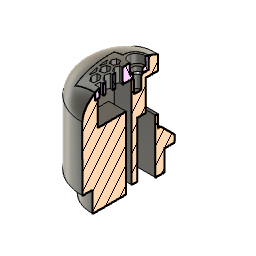
sensorhead_v2_filterBolt v4 (Autodesk Fusion 360 design; units mm, degrees)
Autodesk Fusion 360 part; units mm, degrees
sketch "Sketch1" plane through (0, 0, 0) normal (0, 0, 1) x (1, 0, 0)
  circle A0 centre (0, 0) radius 13
  dimension "d1" = 26
  constraint coincident A0.centre origin
  measures "d1" diameter of A0
extrude "Extrude1" add sketch "Sketch1" along normal blind 7.5 makes body 1
sketch "Sketch2" plane through (0, 0, 7.5) normal (0, 0, 1) x (-1, 0, 0)
  circle A0 centre (0, 0) radius 13
  circle A1 centre (0, 0) radius 16.7
  dimension "d4" = 33.4
  constraint coincident A0.centre A1.centre
  measures "d4" diameter of A1
extrude "Extrude2" add sketch "Sketch2" along normal blind 30 contours A0 | A1 bodies 1
sketch "Sketch8" plane through (0, 0, 0) normal (0, 1, 0) x (1, 0, 0)
  line L0 (0, -37.5) -> (0, -27.5)
  line L1 (16.7, -27.5) -> (0, -27.5)
  line L2 (0, -27.5) -> (0, -37.5)
  ellipse E0 centre (0, -27.5) end of major axis (-16.7, -27.5) minor radius 10 (0, -37.5) -> (16.7, -27.5) ccw
  line L3 (16.7, -27.5) -> (16.7, -37.5)
  line L4 (16.7, -37.5) -> (0, -37.5)
  dimension "d66" = 10
  dimension "d67" = 33.4
  constraint vertical L0
  constraint coincident L0.end L1.end
  constraint perpendicular L1 L3
  constraint perpendicular L3 L4
  measures "d66" distance of L0.start L0.end
  measures "d67" distance of E0
revolve "Revolve1" cut sketch "Sketch8" angle 360 about axis through (0, 0, 27.5) along (0, 0, 1) contours E0 L3 L4 bodies 1
sketch "Sketch3" plane through (0, 0, 0) normal (0, 0, -1) x (1, 0, 0)
  circle A0 centre (0, 0) radius 13
  line L0 (-7.875, -6.2) -> (7.875, -6.2)
  line L1 (7.875, -6.2) -> (7.875, -8.2)
  line L2 (-7.875, -8.2) -> (-7.875, -6.2)
  line L3 (-7.875, -6.2) -> (7.875, -8.2) construction
  line L4 (7.875, -6.2) -> (-7.875, -8.2) construction
  line L5 (6.5, -8.2) -> (6.5, -9.7)
  line L6 (-6.5, -9.7) -> (-6.5, -8.2)
  line L7 (-6.5, -8.2) -> (6.5, -10.2) construction
  line L8 (6.5, -8.2) -> (-6.5, -10.2) construction
  line L9 (-6.5, -6.2) -> (6.5, -6.2)
  line L10 (6.5, -6.2) -> (6.5, -1.2)
  line L11 (6.5, -1.2) -> (-6.5, -1.2)
  line L12 (-6.5, -1.2) -> (-6.5, -6.2)
  line L13 (-6.5, -6.2) -> (6.5, -1.2) construction
  line L14 (6.5, -6.2) -> (-6.5, -1.2) construction
  line L15 (7.875, -8.2) -> (6.5, -8.2)
  line L16 (-6.5, -8.2) -> (-7.875, -8.2)
  line L17 (6.5, -9.7) -> (-6.5, -9.7)
  point P0 (0, -7.2)
  point P1 (0, -9.2)
  point P2 (0, -3.7)
  dimension "d9" = 15.75
  dimension "d10" = 2
  dimension "d13" = 13
  dimension "d15" = 13
  dimension "d132" = 0.5
  constraint horizontal L0
  constraint perpendicular L0 L1
  constraint parallel L0 L15
  constraint parallel L1 L2
  constraint coincident L3 P0
  constraint coincident L4 P0
  constraint parallel L5 L6
  constraint coincident L7 P1
  constraint coincident L8 P1
  constraint horizontal L9
  constraint perpendicular L9 L10
  constraint parallel L9 L11
  constraint parallel L10 L12
  constraint coincident L13 P2
  constraint coincident L14 P2
  constraint collinear L15 L16
  constraint perpendicular L6 L17
  measures "d9" distance of L1.end L2.start
  measures "d10" distance of L0.end L1.end
  measures "d13" distance of L7.end L8.end
  measures "d15" distance of L10.end L11.end
  measures "d132" distance of L7.end L5.end
sketch "Sketch4" plane through (0, 0, 0) normal (1, 0, 0) x (0, 1, 0)
  line L0 (0, 12) -> (10.7, 12)
  line L1 (10.7, 12) -> (21.5887, 12)
  line L2 (21.5887, 12) -> (21.5887, 38.7585)
  line L3 (21.5887, 38.7585) -> (10.7, 38.7585)
  line L4 (10.7, 38.7585) -> (10.7, 12)
  dimension "d17" = 10.7
  constraint horizontal L1
  constraint vertical L2
  constraint horizontal L3
  constraint vertical L4
  measures "d17" distance of L0.start L0.end
sketch "Sketch5" plane through (0, 0, 0) normal (1, 0, 0) x (0, 1, 0)
extrude "Extrude3" cut sketch "Sketch4" along normal blind 26 bodies 1
extrude "Extrude4" cut 1 faces at (0, 12.7, 24.8926) along direction (-1, 0, 0) blind 20 on bodies 1 bodies 1
extrude "Extrude5" cut sketch "Sketch3" against normal blind 30 contours L0 L1 L2 L5 L6 L9 L15 L16 L17 bodies 1
extrude "Extrude6" cut sketch "Sketch3" against normal blind 19 contours L0 L9 L10 L11 L12 bodies 1
sketch "Sketch6" plane through (0, 10.7, 0) normal (0, 1, 0) x (-1, 0, 0)
  line L0 (-12.8219, 27.5) -> (-12.8219, 12)
  line L1 (-12.8219, 12) -> (12.8219, 12)
  line L2 (6.5, 16.5) -> (-6.5, 16.5)
  line L3 (-6.5, 16.5) -> (-6.5, 29.5)
  line L4 (-6.5, 29.5) -> (6.5, 29.5)
  line L5 (6.5, 29.5) -> (6.5, 16.5)
  line L6 (6.5, 16.5) -> (-6.5, 29.5) construction
  line L7 (-6.5, 16.5) -> (6.5, 29.5) construction
  line L8 (12.8219, 12) -> (12.8219, 27.5)
  spline S0 degree 3 poles (0, 35.1778) (0.2245, 35.1778) (0.4491, 35.1742) (1.1338, 35.1527) (1.5943, 35.1233) (2.7541, 35.0106) (3.4543, 34.9068) (5.6711, 34.4534) (7.1958, 33.9489) (9.6653, 32.6226) (10.586, 31.9216) (11.7837, 30.5905) (12.1987, 29.9679) (12.6993, 28.7104) (12.8219, 28.1132) (12.8219, 27.5) knots -1.453792 -1.453792 -1.453792 -1.453792 -1.397904 -1.397904 -1.283214 -1.283214 -1.107738 -1.107738 -0.719665 -0.719665 -0.405775 -0.405775 -0.183953 -0.183953 0 0 0 0
  spline S1 degree 3 poles (-12.8219, 27.5) (-12.8219, 27.8392) (-12.7843, 28.1754) (-12.6354, 28.8496) (-12.5226, 29.1821) (-12.055, 30.2186) (-11.5805, 30.8593) (-10.1007, 32.3522) (-8.8544, 33.1585) (-6.5098, 34.1443) (-5.6112, 34.4282) (-3.9195, 34.8277) (-3.1196, 34.963) (-1.813, 35.1068) (-1.3053, 35.1439) (-0.532, 35.1728) (-0.266, 35.1778) (0, 35.1778) knots -1.833651 -1.833651 -1.833651 -1.833651 -1.708322 -1.708322 -1.578523 -1.578523 -1.288251 -1.288251 -0.803835 -0.803835 -0.524093 -0.524093 -0.282154 -0.282154 -0.129741 -0.129741 -0.04999 -0.04999 -0.04999 -0.04999
  point P0 (0, 23)
  dimension "d26" = 13
  dimension "d27" = 13
  constraint horizontal L2
  constraint perpendicular L2 L3
  constraint parallel L2 L4
  constraint parallel L3 L5
  constraint coincident L6 P0
  constraint coincident L7 P0
  measures "d26" distance of L3.end L4.end
  measures "d27" distance of L2.end L3.end
extrude "Extrude7" cut sketch "Sketch6" against normal blind 1 contours L2 L3 L4 L5 bodies 1
extrude "Extrude8" cut 1 faces at (2.1667, 10.3667, 29.5) along direction (0, 0, 1) blind 0.5 on bodies 1 bodies 1
ref_plane "WorkPlane1" through (0, 0, 40) normal (0, 0, 1) x (1, 0, 0)
sketch "Sketch7" plane through (0, 0, 40) normal (0, 0, 1) x (1, 0, 0)
  line L0 (7, 2) -> (7, -12)
  line L1 (7, -12) -> (-7, -12)
  line L2 (-7, -12) -> (-7, 2)
  line L3 (-7, 2) -> (7, -12) construction
  line L4 (7, 2) -> (-7, -12) construction
  line L5 (7.125, 2.125) -> (7.125, -12.125)
  line L6 (7.125, -12.125) -> (-7.125, -12.125)
  line L7 (-7.125, -12.125) -> (-7.125, 2.125)
  line L8 (-7.125, 2.125) -> (7.125, -12.125) construction
  line L9 (7.125, 2.125) -> (-7.125, -12.125) construction
  line L10 (-4, 2.125) -> (-4, 3.325)
  line L11 (4, 2.125) -> (4, 3.325)
  line L12 (-7.125, 2.125) -> (-4, 2.125)
  line L13 (4, 2.125) -> (7.125, 2.125)
  arc A0 (4, 3.325) -> (-4, 3.325) centre (0, 3.325) ccw
  line L14 (-4, 2) -> (-3.9, 2)
  line L15 (-3.9, 2) -> (-3.9, 3.325)
  line L16 (4, 2) -> (3.9, 2)
  line L17 (3.9, 2) -> (3.9, 3.325)
  arc A1 (3.9, 3.325) -> (-3.9, 3.325) centre (0, 3.325) ccw
  line L18 (-7, 2) -> (-3.9, 2)
  line L19 (3.9, 2) -> (7, 2)
  circle A2 centre (0, 3.325) radius 1.35
  circle A3 centre (0, 3.325) radius 2.1
  circle A4 centre (0, 3.325) radius 1.75
  circle A5 centre (0, 3.325) radius 2.875
  point P0 (0, -5)
  point P1 (0, -5)
  dimension "d35" = 14.25
  dimension "d36" = 14.25
  dimension "d135" = 7.8
  dimension "d136" = 0.1
  dimension "d137" = 0.1
  dimension "d138" = 2.7
  dimension "d139" = 4.2
  dimension "d140" = 3.5
  dimension "d141" = 5.75
  constraint horizontal L18
  constraint perpendicular L0 L18
  constraint parallel L1 L18
  constraint parallel L0 L2
  constraint coincident L3 P1
  constraint coincident L4 P1
  constraint horizontal L12
  constraint perpendicular L5 L12
  constraint parallel L6 L12
  constraint parallel L5 L7
  constraint coincident L8 P1
  constraint coincident L9 P1
  constraint coincident P1 P0
  constraint vertical L10
  constraint collinear L12 L13
  constraint concentric A0 A1
  constraint coincident L14.start L18
  constraint parallel L14 L18
  constraint tangent L15 A1
  constraint perpendicular L15 L18
  constraint coincident L16.start L18
  constraint perpendicular L11 L16
  constraint vertical L17
  constraint tangent L17 A1
  constraint collinear L18 L19
  constraint concentric A0 A2
  constraint concentric A1 A3
  constraint concentric A2 A4
  constraint concentric A2 A5
  measures "d35" distance of L5.end L6.end
  measures "d36" distance of L5.start L5.end
  measures "d135" diameter of A1
  measures "d136" distance of L14.start L14.end
  measures "d137" distance of L16.start L16.end
  measures "d138" diameter of A2
  measures "d139" diameter of A3
  measures "d140" diameter of A4
  measures "d141" diameter of A5
copy_body "Body->Comp1" bodies 1 removing the originals makes body 2 in component "sensorHead"
extrude "Extrude11" add 1 faces at (15.4266, 0, 7.5) along direction (0, 0, -1) blind 3 on bodies 2 bodies 2 in component "sensorHead"
sketch "Sketch2 (2)" plane through (0, 0, 0) normal (1, 0, 0) x (0, 1, 0) in component "sensorHead"
  line L0 (10.7, 12) -> (16.7, 12)
  line L1 (-16.7, 4.5) -> (16.7, 4.5)
  line L2 (16.7, 12) -> (16.7, 4.5)
  line L3 (10.7, 12) -> (11.7, 12)
  line L4 (11.7, 12) -> (16.7, 7)
  line L5 (16.7, 12) -> (11.7, 12)
  point P0 (10.7, 12)
  dimension "d157" = 1
  dimension "d158" = 45
  constraint coincident L0.end L2.start
  constraint coincident L1.end L2.end
  constraint coincident P0 L0.start
  constraint coincident L0 L3.end
  constraint coincident L2 L4.end
  measures "d157" distance of P0 L3.end
  measures "d158" angle of L3 L4
extrude "Extrude5'" cut sketch "Sketch2 (2)" along normal mid plane 33 bodies 2 in component "sensorHead"
extrude "Extrude12" add 1 faces at (0.3238, -3.5212, 0) along direction (0, 0, -1) blind 3 on bodies 2 bodies 2 in component "sensorHead"
extrude "Extrude1'" cut sketch "Sketch7" against normal blind 8 contours L0 L1 L2 L14 L15 L16 L17 A1 L18 L19 | L5 L6 L7 L10 L11 L12 L13 A0 | A2 | A3 | A4 | A5 bodies 2 in component "sensorHead"
sketch "Sketch1 (2)" plane through (0, 0, 32) normal (0, 0, 1) x (-1, 0, 0) in component "sensorHead"
  line L0 (7.125, 12.125) -> (-7.125, 12.125)
  line L1 (-7.125, 12.125) -> (-7.125, -2.125)
  line L2 (4, -2.125) -> (7.125, -2.125)
  line L3 (7.125, -2.125) -> (7.125, 12.125)
  line L4 (6.125, -1.125) -> (-6.125, -1.125)
  line L5 (-6.125, -1.125) -> (-6.125, 11.125)
  line L6 (-6.125, 11.125) -> (6.125, 11.125)
  line L7 (6.125, 11.125) -> (6.125, -1.125)
  line L8 (6.125, -1.125) -> (-6.125, 11.125) construction
  line L9 (-6.125, -1.125) -> (6.125, 11.125) construction
  line L10 (-6.125, -1.125) -> (6.125, -1.125)
  line L11 (6.125, -1.125) -> (6.125, 0.875)
  line L12 (6.125, 0.875) -> (-6.125, 0.875)
  line L13 (-6.125, 0.875) -> (-6.125, -1.125)
  arc A0 (-4, -3.325) -> (4, -3.325) centre (0, -3.325) ccw
  line L14 (4, -3.325) -> (4, -2.125)
  line L15 (-7.125, -2.125) -> (-4, -2.125)
  line L16 (-4, -2.125) -> (-4, -3.325)
  point P0 (0, 5)
  dimension "d39" = 12.25
  dimension "d40" = 12.25
  dimension "d41" = 12.25
  dimension "d42" = 2
  constraint horizontal L4
  constraint perpendicular L4 L5
  constraint parallel L4 L6
  constraint parallel L5 L7
  constraint coincident L8 P0
  constraint coincident L9 P0
  constraint horizontal L10
  constraint vertical L11
  constraint horizontal L12
  constraint vertical L13
  measures "d39" distance of L5.end L6.end
  measures "d40" distance of L4.end L5.end
  measures "d41" distance of L4.end L4.start
  measures "d42" distance of L4.end L12.end
extrude "Extrude2'" cut sketch "Sketch1 (2)" against normal blind 47 contours L4 L5 L7 L10 L11 L12 L13 bodies 2 in component "sensorHead"
extrude "Extrude3'" add 2 faces at (2.1667, 1.2, -1) (2.1667, 1.2, 6.3333) along direction (0, 1, 0) blind 1.925 on bodies 2 bodies 2 in component "sensorHead"
extrude "Extrude4'" cut sketch "Sketch1 (2)" against normal blind 6 contours L5 L6 L7 L12 bodies 2 in component "sensorHead"
extrude "Extrude9" add sketch "Sketch7" against normal blind 7.9 separate body contours L0 L1 L2 L14 L15 L16 L17 A1 L18 L19 | A2 | A3 | A4 | A5 makes body 3
revolve "Revolve2" cut sketch "Sketch8" angle 360 about axis through (0, 0, 37.5) along (0, 0, -1) contours L0 L1 L2 E0 keep common part bodies 3
sketch "Sketch9" plane through (0, 0, 32.1) normal (0, 0, -1) x (1, 0, 0)
  line L0 (7, 12) -> (-7, 12)
  line L1 (-7, 12) -> (-7, -2)
  line L2 (3.9, -2) -> (7, -2)
  line L3 (7, -2) -> (7, 12)
  line L4 (7, -2) -> (-7, -2)
  line L5 (-7, -2) -> (-7, 12)
  line L6 (-7, 12) -> (7, 12)
  line L7 (7, 12) -> (7, -2)
  line L8 (-5.5, 10.5) -> (5.5, 10.5)
  line L9 (5.5, 10.5) -> (5.5, -0.5)
  line L10 (5.5, -0.5) -> (-5.5, -0.5)
  line L11 (-5.5, -0.5) -> (-5.5, 10.5)
  line L12 (1.5, -0.0043) -> (0.7537, 1.2969)
  line L13 (0.7537, 1.2969) -> (-0.7463, 1.3012)
  line L14 (-0.7463, 1.3012) -> (-1.5, 0.0043)
  line L15 (-1.5, 0.0043) -> (-0.7537, -1.2969)
  line L16 (-0.7537, -1.2969) -> (0.7463, -1.3012)
  line L17 (0.7463, -1.3012) -> (1.5, -0.0043)
  line L18 (-5.2537, -1.3012) -> (-4.5, -0.0043)
  line L19 (-6.7537, -1.2969) -> (-5.2537, -1.3012)
  line L20 (-7.5, 0.0043) -> (-6.7537, -1.2969)
  line L21 (-6.7463, 1.3012) -> (-7.5, 0.0043)
  line L22 (-5.2463, 1.2969) -> (-6.7463, 1.3012)
  line L23 (-4.5, -0.0043) -> (-5.2463, 1.2969)
  line L24 (6.7463, -1.3012) -> (7.5, -0.0043)
  line L25 (5.2463, -1.2969) -> (6.7463, -1.3012)
  line L26 (4.5, 0.0043) -> (5.2463, -1.2969)
  line L27 (5.2537, 1.3012) -> (4.5, 0.0043)
  line L28 (6.7537, 1.2969) -> (5.2537, 1.3012)
  line L29 (7.5, -0.0043) -> (6.7537, 1.2969)
  line L30 (-5.2537, 2.1988) -> (-4.5, 3.4957)
  line L31 (-6.7537, 2.2031) -> (-5.2537, 2.1988)
  line L32 (-7.5, 3.5043) -> (-6.7537, 2.2031)
  line L33 (-6.7463, 4.8012) -> (-7.5, 3.5043)
  line L34 (-5.2463, 4.7969) -> (-6.7463, 4.8012)
  line L35 (-4.5, 3.4957) -> (-5.2463, 4.7969)
  line L36 (0.7463, 2.1988) -> (1.5, 3.4957)
  line L37 (-0.7537, 2.2031) -> (0.7463, 2.1988)
  line L38 (-1.5, 3.5043) -> (-0.7537, 2.2031)
  line L39 (-0.7463, 4.8012) -> (-1.5, 3.5043)
  line L40 (0.7537, 4.7969) -> (-0.7463, 4.8012)
  line L41 (1.5, 3.4957) -> (0.7537, 4.7969)
  line L42 (6.7463, 2.1988) -> (7.5, 3.4957)
  line L43 (5.2463, 2.2031) -> (6.7463, 2.1988)
  line L44 (4.5, 3.5043) -> (5.2463, 2.2031)
  line L45 (5.2537, 4.8012) -> (4.5, 3.5043)
  line L46 (6.7537, 4.7969) -> (5.2537, 4.8012)
  line L47 (7.5, 3.4957) -> (6.7537, 4.7969)
  line L48 (-5.2537, 5.6988) -> (-4.5, 6.9957)
  line L49 (-6.7537, 5.7031) -> (-5.2537, 5.6988)
  line L50 (-7.5, 7.0043) -> (-6.7537, 5.7031)
  line L51 (-6.7463, 8.3012) -> (-7.5, 7.0043)
  line L52 (-5.2463, 8.2969) -> (-6.7463, 8.3012)
  line L53 (-4.5, 6.9957) -> (-5.2463, 8.2969)
  line L54 (0.7463, 5.6988) -> (1.5, 6.9957)
  line L55 (-0.7537, 5.7031) -> (0.7463, 5.6988)
  line L56 (-1.5, 7.0043) -> (-0.7537, 5.7031)
  line L57 (-0.7463, 8.3012) -> (-1.5, 7.0043)
  line L58 (0.7537, 8.2969) -> (-0.7463, 8.3012)
  line L59 (1.5, 6.9957) -> (0.7537, 8.2969)
  line L60 (6.7463, 5.6988) -> (7.5, 6.9957)
  line L61 (5.2463, 5.7031) -> (6.7463, 5.6988)
  line L62 (4.5, 7.0043) -> (5.2463, 5.7031)
  line L63 (5.2537, 8.3012) -> (4.5, 7.0043)
  line L64 (6.7537, 8.2969) -> (5.2537, 8.3012)
  line L65 (7.5, 6.9957) -> (6.7537, 8.2969)
  line L66 (-5.2537, 9.1988) -> (-4.5, 10.4957)
  line L67 (-6.7537, 9.2031) -> (-5.2537, 9.1988)
  line L68 (-7.5, 10.5043) -> (-6.7537, 9.2031)
  line L69 (-6.7463, 11.8012) -> (-7.5, 10.5043)
  line L70 (-5.2463, 11.7969) -> (-6.7463, 11.8012)
  line L71 (-4.5, 10.4957) -> (-5.2463, 11.7969)
  line L72 (0.7463, 9.1988) -> (1.5, 10.4957)
  line L73 (-0.7537, 9.2031) -> (0.7463, 9.1988)
  line L74 (-1.5, 10.5043) -> (-0.7537, 9.2031)
  line L75 (-0.7463, 11.8012) -> (-1.5, 10.5043)
  line L76 (0.7537, 11.7969) -> (-0.7463, 11.8012)
  line L77 (1.5, 10.4957) -> (0.7537, 11.7969)
  line L78 (6.7463, 9.1988) -> (7.5, 10.4957)
  line L79 (5.2463, 9.2031) -> (6.7463, 9.1988)
  line L80 (4.5, 10.5043) -> (5.2463, 9.2031)
  line L81 (5.2537, 11.8012) -> (4.5, 10.5043)
  line L82 (6.7537, 11.7969) -> (5.2537, 11.8012)
  line L83 (7.5, 10.4957) -> (6.7537, 11.7969)
  line L84 (3.7463, -3.2012) -> (4.5, -1.9043)
  line L85 (4.5, -1.9043) -> (3.7537, -0.6031)
  line L86 (3.7537, -0.6031) -> (2.2537, -0.5988)
  line L87 (2.2537, -0.5988) -> (1.5, -1.8957)
  line L88 (1.5, -1.8957) -> (2.2463, -3.1969)
  line L89 (2.2463, -3.1969) -> (3.7463, -3.2012)
  line L90 (-1.5, -1.9043) -> (-2.2463, -0.6031)
  line L91 (-2.2463, -0.6031) -> (-3.7463, -0.5988)
  line L92 (-3.7463, -0.5988) -> (-4.5, -1.8957)
  line L93 (-4.5, -1.8957) -> (-3.7537, -3.1969)
  line L94 (-3.7537, -3.1969) -> (-2.2537, -3.2012)
  line L95 (-2.2537, -3.2012) -> (-1.5, -1.9043)
  line L96 (-7.5, -1.9043) -> (-8.2463, -0.6031)
  line L97 (-8.2463, -0.6031) -> (-9.7463, -0.5988)
  line L98 (-9.7463, -0.5988) -> (-10.5, -1.8957)
  line L99 (-10.5, -1.8957) -> (-9.7537, -3.1969)
  line L100 (-9.7537, -3.1969) -> (-8.2537, -3.2012)
  line L101 (-8.2537, -3.2012) -> (-7.5, -1.9043)
  line L102 (4.5, 1.6582) -> (3.7537, 2.9594)
  line L103 (3.7537, 2.9594) -> (2.2537, 2.9637)
  line L104 (2.2537, 2.9637) -> (1.5, 1.6668)
  line L105 (1.5, 1.6668) -> (2.2463, 0.3656)
  line L106 (2.2463, 0.3656) -> (3.7463, 0.3613)
  line L107 (3.7463, 0.3613) -> (4.5, 1.6582)
  line L108 (-1.5, 1.6582) -> (-2.2463, 2.9594)
  line L109 (-2.2463, 2.9594) -> (-3.7463, 2.9637)
  line L110 (-3.7463, 2.9637) -> (-4.5, 1.6668)
  line L111 (-4.5, 1.6668) -> (-3.7537, 0.3656)
  line L112 (-3.7537, 0.3656) -> (-2.2537, 0.3613)
  line L113 (-2.2537, 0.3613) -> (-1.5, 1.6582)
  line L114 (-7.5, 1.6582) -> (-8.2463, 2.9594)
  line L115 (-8.2463, 2.9594) -> (-9.7463, 2.9637)
  line L116 (-9.7463, 2.9637) -> (-10.5, 1.6668)
  line L117 (-10.5, 1.6668) -> (-9.7537, 0.3656)
  line L118 (-9.7537, 0.3656) -> (-8.2537, 0.3613)
  line L119 (-8.2537, 0.3613) -> (-7.5, 1.6582)
  line L120 (4.5, 5.2207) -> (3.7537, 6.5219)
  line L121 (3.7537, 6.5219) -> (2.2537, 6.5262)
  line L122 (2.2537, 6.5262) -> (1.5, 5.2293)
  line L123 (1.5, 5.2293) -> (2.2463, 3.9281)
  line L124 (2.2463, 3.9281) -> (3.7463, 3.9238)
  line L125 (3.7463, 3.9238) -> (4.5, 5.2207)
  line L126 (-1.5, 5.2207) -> (-2.2463, 6.5219)
  line L127 (-2.2463, 6.5219) -> (-3.7463, 6.5262)
  line L128 (-3.7463, 6.5262) -> (-4.5, 5.2293)
  line L129 (-4.5, 5.2293) -> (-3.7537, 3.9281)
  line L130 (-3.7537, 3.9281) -> (-2.2537, 3.9238)
  line L131 (-2.2537, 3.9238) -> (-1.5, 5.2207)
  line L132 (-7.5, 5.2207) -> (-8.2463, 6.5219)
  line L133 (-8.2463, 6.5219) -> (-9.7463, 6.5262)
  line L134 (-9.7463, 6.5262) -> (-10.5, 5.2293)
  line L135 (-10.5, 5.2293) -> (-9.7537, 3.9281)
  line L136 (-9.7537, 3.9281) -> (-8.2537, 3.9238)
  line L137 (-8.2537, 3.9238) -> (-7.5, 5.2207)
  line L138 (4.5, 8.7832) -> (3.7537, 10.0844)
  line L139 (3.7537, 10.0844) -> (2.2537, 10.0887)
  line L140 (2.2537, 10.0887) -> (1.5, 8.7918)
  line L141 (1.5, 8.7918) -> (2.2463, 7.4906)
  line L142 (2.2463, 7.4906) -> (3.7463, 7.4863)
  line L143 (3.7463, 7.4863) -> (4.5, 8.7832)
  line L144 (-1.5, 8.7832) -> (-2.2463, 10.0844)
  line L145 (-2.2463, 10.0844) -> (-3.7463, 10.0887)
  line L146 (-3.7463, 10.0887) -> (-4.5, 8.7918)
  line L147 (-4.5, 8.7918) -> (-3.7537, 7.4906)
  line L148 (-3.7537, 7.4906) -> (-2.2537, 7.4863)
  line L149 (-2.2537, 7.4863) -> (-1.5, 8.7832)
  line L150 (-7.5, 8.7832) -> (-8.2463, 10.0844)
  line L151 (-8.2463, 10.0844) -> (-9.7463, 10.0887)
  line L152 (-9.7463, 10.0887) -> (-10.5, 8.7918)
  line L153 (-10.5, 8.7918) -> (-9.7537, 7.4906)
  line L154 (-9.7537, 7.4906) -> (-8.2537, 7.4863)
  line L155 (-8.2537, 7.4863) -> (-7.5, 8.7832)
  line L156 (4.5, 12.3457) -> (3.7537, 13.6469)
  line L157 (3.7537, 13.6469) -> (2.2537, 13.6512)
  line L158 (2.2537, 13.6512) -> (1.5, 12.3543)
  line L159 (1.5, 12.3543) -> (2.2463, 11.0531)
  line L160 (2.2463, 11.0531) -> (3.7463, 11.0488)
  line L161 (3.7463, 11.0488) -> (4.5, 12.3457)
  line L162 (-1.5, 12.3457) -> (-2.2463, 13.6469)
  line L163 (-2.2463, 13.6469) -> (-3.7463, 13.6512)
  line L164 (-3.7463, 13.6512) -> (-4.5, 12.3543)
  line L165 (-4.5, 12.3543) -> (-3.7537, 11.0531)
  line L166 (-3.7537, 11.0531) -> (-2.2537, 11.0488)
  line L167 (-2.2537, 11.0488) -> (-1.5, 12.3457)
  line L168 (-7.5, 12.3457) -> (-8.2463, 13.6469)
  line L169 (-8.2463, 13.6469) -> (-9.7463, 13.6512)
  line L170 (-9.7463, 13.6512) -> (-10.5, 12.3543)
  line L171 (-10.5, 12.3543) -> (-9.7537, 11.0531)
  line L172 (-9.7537, 11.0531) -> (-8.2537, 11.0488)
  line L173 (-8.2537, 11.0488) -> (-7.5, 12.3457)
  arc A0 (-3.9, -3.325) -> (3.9, -3.325) centre (0, -3.325) ccw
  line L174 (3.9, -3.325) -> (3.9, -2)
  line L175 (-7, -2) -> (-3.9, -2)
  line L176 (-3.9, -2) -> (-3.9, -3.325)
  dimension "d75" = 1.5
  dimension "d76" = 1.5
  dimension "d79" = 6
  dimension "d80" = 10.5
  dimension "d95" = -12
  dimension "d96" = 14.25
  constraint horizontal L4
  constraint vertical L5
  constraint horizontal L6
  constraint vertical L7
  constraint coincident L0.end L1.start
  constraint coincident L2.end L3.start
  measures "d76" distance of L12.start origin
extrude "Extrude12'" cut sketch "Sketch9" against normal blind 12 contours L9 L61 L62 L63 L64 | L8 L72 L73 L74 L77 | L9 L43 L44 L45 L46 | L11 L48 L49 L52 L53 | L11 L30 L31 L34 L35 | L36 L37 L38 L39 L40 L41 | L54 L55 L56 L57 L58 L59 | L102 L103 L104 L105 L106 L107 | L108 L109 L110 L111 L112 L113 | L120 L121 L122 L123 L124 L125 | L126 L127 L128 L129 L130 L131 | L138 L139 L140 L141 L142 L143 | L144 L145 L146 L147 L148 L149 bodies 3
extrude "Extrude8'" cut 1 faces at (-2.0417, -4.2917, 26) along direction (0, 0, -1) blind 3 on bodies 2 bodies 2 in component "sensorHead"
extrude "Extrude13" cut sketch "Sketch7" against normal blind 6.2 contours A2 | A3 | A4 | A5 bodies 3
extrude "Extrude14" cut sketch "Sketch7" against normal blind 12 contours A2 | A4 bodies 3
extrude "Extrude17" cut sketch "Sketch7" against normal blind 5 from surface at -8 contours A2 bodies 2 in component "sensorHead"
chamfer "Chamfer2" distance 0.5 angle 45 1 edges at (-1.2586, 3.8132, 32) on bodies 2 in component "sensorHead"
sketch "Sketch12" plane through (0, 0, -3) normal (0, 0, -1) x (1, 0, 0)
  line L0 (6.125, -1.125) -> (-6.125, -1.125)
  line L1 (-6.125, -1.125) -> (-6.125, 0.875)
  line L2 (-6.125, 0.875) -> (6.125, 0.875)
  line L3 (6.125, 0.875) -> (6.125, -1.125)
  circle A0 centre (0, 0) radius 13
  line L4 (-6.5, -6.2) -> (-6.5, -3.125)
  line L5 (-6.5, -3.125) -> (6.5, -3.125)
  line L6 (6.5, -3.125) -> (6.5, -6.2)
  line L7 (6.5, -6.2) -> (7.875, -6.2)
  line L8 (7.875, -6.2) -> (7.875, -8.2)
  line L9 (7.875, -8.2) -> (6.5, -8.2)
  line L10 (6.5, -8.2) -> (6.5, -9.7)
  line L11 (6.5, -9.7) -> (-6.5, -9.7)
  line L12 (-6.5, -9.7) -> (-6.5, -8.2)
  line L13 (-6.5, -8.2) -> (-7.875, -8.2)
  line L14 (-7.875, -8.2) -> (-7.875, -6.2)
  line L15 (-7.875, -6.2) -> (-6.5, -6.2)
  line L16 (-6.5, -3.125) -> (-6.125, -1.125)
  line L17 (6.5, -3.125) -> (6.125, -1.125)
  line L18 (-6.5, -3.125) -> (6.5, -3.125)
  line L19 (6.125, -1.125) -> (-6.125, -1.125)
  constraint coincident L4.end L5.start
  constraint coincident L0.end L1.start
  constraint coincident L5.end L6.start
  constraint coincident L0.start L3.end
extrude "Extrude19" cut sketch "Sketch12" against normal blind 2 contours L0 L5 L16 L17 L18 L19 bodies 2 in component "sensorHead"
extrude "Extrude18" [suppressed] in component "sensorHead"
component "sensorHead" placed x (1, 0, 0) y (0, 1, 0) z (0, 0, 1) at (0, 0, 0)
